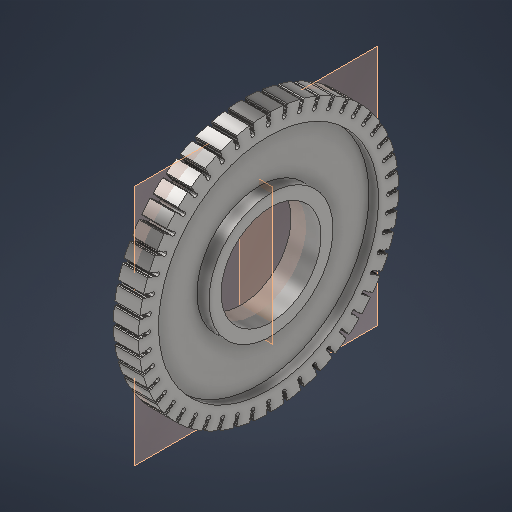
# Autodesk Inventor part: DiscoPaleStadio6-DimensioniAprossimate
Saved by Autodesk Inventor 2026.2 (Build 302298010, 298A)
## iProperties
Created: 2026-04-19
Part Number: DiscoPaleStadio6-DimensioniAprossimate
Material: Steel, Alloy
Document SubType Name: Modeling
Designer: Yan
Density: 7.73 g/cm^3
Appearance: Semi-Polished
Author: Yan
Autodesk Inventor part; units mm, degrees
ref_plane "XZ Plane" through (0, 0, 0) normal (0, 1, 0) x (-1, 0, 0)
sketch "Sketch1" plane through (0, 0, 0) normal (1, 0, 0) x (0, 1, 0)
  circle A0 centre (0, 0) radius 50
  circle A1 centre (0, 0) radius 62
  dimension "d0" = 100
  dimension "d1" = 124
  constraints: 2 centre point, 2 coincident
  measures "d0" diameter of A0
  measures "d1" diameter of A1
extrude "Extrusion1" add sketch "Sketch1" along normal blind 30
ref_plane "Work Plane1" through (0, 0, 0) normal (0, 0, 1) x (1, 0, 0)
sketch "Sketch2" plane through (0, 0, 0) normal (0, 0, 1) x (1, 0, 0)
  line L0 (0, 62) -> (30, 62) projected
  line L1 (18, 62) -> (18, 110)
  line L2 (18, 110) -> (12, 110)
  line L3 (12, 110) -> (12, 62)
  line L4 (0, -62) -> (0, 62) projected
  line L5 (-6, 0) -> (36, 0) projected
  point P0 (0, 0)
  dimension "d5" = 6
  dimension "d6" = 12
  dimension "d7" = 48
  constraints: 6 end point, 3 perpendicular, 2 point on line
  measures "d5" distance between parallel lines of L3 L1
  measures "d6" distance between parallel lines of L4 L3
  measures "d7" distance between parallel lines of L0 L2
revolve "Revolution1" add sketch "Sketch2" angle 360 about axis through (-10, 0, 0) along (1, 0, 0)
ref_plane "Work Plane2" through (15, 0, 0) normal (1, 0, 0) x (0, 1, 0)
sketch "Sketch3" plane through (15, 0, 0) normal (1, 0, 0) x (0, 1, 0)
  circle A0 centre (0, 0) radius 130
  circle A1 centre (0, 0) radius 110
  dimension "d10" = 260
  dimension "d11" = 220
  constraints: 2 centre point, 2 coincident
  measures "d10" diameter of A0
  measures "d11" diameter of A1
extrude "Extrusion2" add sketch "Sketch3" along normal mid plane 25
sketch "Sketch4" plane through (27.5, 0, 0) normal (1, 0, 0) x (0, 0, -1)
  line L0 (-2.1774, 130) -> (-1.6, 129)
  line L1 (-1.6, 129) -> (-1.6, 128)
  line L2 (-1.6, 128) -> (-2, 127.3072)
  line L3 (-2, 127.3072) -> (-2, 126.3072)
  line L4 (-2, 126.3072) -> (-1.3, 125.0947)
  line L5 (-1.3, 125.0947) -> (-1.3, 124.0947)
  line L6 (-1.3, 124.0947) -> (-1.6, 123.5751)
  line L7 (-1.6, 123.5751) -> (-1.6, 122.5751)
  line L8 (-1.6, 122.5751) -> (-1.3, 122.0555)
  line L9 (-1.3, 122.0555) -> (-1.3, 121.5199)
  line L10 (0, 130) -> (0, 120)
  line L11 (2.1774, 130) -> (1.6, 129)
  line L12 (1.6, 129) -> (1.6, 128)
  line L13 (1.6, 128) -> (2, 127.3072)
  line L14 (2, 127.3072) -> (2, 126.3072)
  line L15 (2, 126.3072) -> (1.3, 125.0947)
  line L16 (1.3, 125.0947) -> (1.3, 124.0947)
  line L17 (1.3, 124.0947) -> (1.6, 123.5751)
  line L18 (1.6, 123.5751) -> (1.6, 122.5751)
  line L19 (1.6, 122.5751) -> (1.3, 122.0555)
  line L20 (1.3, 122.0555) -> (1.3, 121.5199)
  line L21 (-2.1774, 130) -> (2.1774, 130)
  arc A0 (-1.3, 121.5199) -> (1.3, 121.5199) centre (0, 120) ccw
  point P0 (0, 0)
  dimension "d14" = 1.6
  dimension "d15" = 2
  dimension "d16" = 1.3
  dimension "d17" = 1.6
  dimension "d18" = 2
  dimension "d19" = 1
  dimension "d20" = 1
  dimension "d21" = 1
  dimension "d22" = 1
  dimension "d23" = 10
  dimension "d24" = 30
  dimension "d26" = 30
  dimension "d27" = 30
  dimension "d28" = 30
  dimension "d29" = 130
  dimension "d32" = 0
  dimension "d39" = 1
  dimension "d40" = 12
  dimension "d41" = 0
  constraints: 44 end point, 11 symmetric about line, 5 vertical, 2 parallel, 2 point on circle, 2 point on line, 1 centre point, 1 horizontal
  measures "d14" distance between parallel lines of L10 L1
  measures "d15" distance between parallel lines of L10 L3
  measures "d16" distance between parallel lines of L10 L5
  measures "d17" distance between parallel lines of L10 L7
  measures "d18" radius of A0
  measures "d19" vertical distance of L0.start L1.start
  measures "d20" distance of L1.start L1.end
  measures "d21" distance of L3.start L3.end
  measures "d22" distance of L6.end L7.end
  measures "d23" distance of L10.start L10.end
  measures "d24" angle of L10 L6
  measures "d26" angle of L10 L4
  measures "d27" angle of L10 L0
  measures "d28" angle of L10 L2
  measures "d29" distance from line of point (0, 0) L21
  measures "d32" distance from line of point (0, 0) L10
  measures "d39" distance of L4.end L5.end
  measures "d41" distance from line of L21 L10.start
extrude "Extrusion3" cut sketch "Sketch4" against normal through all
pattern_circular "Circular Pattern1" count 48 over 360 about axis through (-10, 0, 0) along (1, 0, 0) of "Extrusion3"
body "Solid1"
